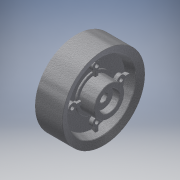
# Autodesk Inventor part: Wheel Hub
Saved by Autodesk Inventor 2018 (Build 220112000, 112)
## iProperties
Created: 2018-08-07
Part Number: Wheel Hub
Material: Generic
Document SubType Name: Modeling
Designer: ruben
Density: 1 g/cm^3
Appearance: Aluminum Cast
Author: ruben
Autodesk Inventor part; units mm, degrees
ref_plane "YZ Plane" through (0, 0, 0) normal (1, 0, 0) x (0, 1, 0)
ref_plane "XZ Plane" through (0, 0, 0) normal (0, 1, 0) x (-1, 0, 0)
ref_plane "XY Plane" through (0, 0, 0) normal (0, 0, 1) x (1, 0, 0)
sketch "Sketch1" plane through (0, 0, 0) normal (0, 1, 0) x (-1, 0, 0)
  line L0 (4.1, 0) -> (-63.1, 0) projected
  line L1 (0, -46.1961) -> (0, 46.6819) projected
  line L2 (-13, -25) -> (-19.5, -25)
  line L3 (-19.5, 25) -> (-13, 25)
  line L4 (-23.9524, -4) -> (-41, -4)
  line L5 (-41, -4) -> (-44, -15)
  line L6 (-23.9524, 4) -> (-41, 4)
  line L7 (-41, 4) -> (-44, 15)
  line L8 (-44, -15) -> (-53.5, -18)
  line L9 (-44, 15) -> (-53.5, 18)
  line L10 (-53.5, -18) -> (-53.5, 18)
  line L11 (-19.5, -25) -> (-19.9524, -6)
  line L12 (-19.9524, 6) -> (-19.5, 25)
  line L13 (-5.5, -16.9) -> (-5.5, 16.9)
  line L14 (-13, -16.9) -> (-5.5, -16.9)
  line L15 (-5.5, 16.9) -> (-13, 16.9)
  line L16 (-13, -25) -> (-13, -16.9)
  line L17 (-13, 16.9) -> (-13, 25)
  line L18 (-44, -26.4766) -> (-44, 27.3254) construction
  line L19 (-19.5, -32.9278) -> (-19.5, 33.4136) construction
  line L20 (-19.9524, -6) -> (-23.9524, -6)
  line L21 (-23.9524, -6) -> (-23.9524, -4)
  line L22 (-23.9524, 4) -> (-23.9524, 6)
  line L23 (-23.9524, 6) -> (-19.9524, 6)
  line L24 (-19.9524, -10.0767) -> (-19.9524, 10.6665) construction
  dimension "d0" = 50
  dimension "d14" = 3
  dimension "d15" = 3
  dimension "d18" = 11
  dimension "d19" = 33.8
  dimension "d36" = 26
  dimension "d48" = 21
  dimension "d49" = 107
  dimension "d50" = 88
  dimension "d52" = 39
  dimension "d53" = 7
  dimension "d54" = 4
  dimension "d56" = 2
  dimension "d57" = 2
  dimension "d58" = 4
  dimension "d60" = 21.0476
  dimension "d61" = 39.9048
  constraints: 46 end point, 10 parallel, 6 point on line, 4 perpendicular, 4 vertical, 2 symmetric about line, 1 collinear, 1 horizontal, 3 other
  measures "d0" distance of L2.start L3.end
  measures "d14" vertical distance of L7.end L9.end
  measures "d15" vertical distance of L5.end L8.end
  measures "d18" diameter of L13 L1
  measures "d19" distance between parallel lines of L15 L14
  measures "d36" diameter of L16 L1
  measures "d48" distance between parallel lines of L4 L2
  measures "d49" diameter of L10 L1
  measures "d50" diameter of L18 L1
  measures "d52" diameter of L19 L1
  measures "d53" distance from line of L2 L8.end
  measures "d54" distance of L11.end L20.end
  measures "d56" distance between parallel lines of L4 L20
  measures "d57" distance of L6.start L22.end
  measures "d58" distance of L12.start L22.end
  measures "d60" horizontal distance of L4.end L11.end
  measures "d61" diameter of L24 L1
revolve "Revolution1" add sketch "Sketch1" angle 360 about axis through (0, 0, -10) along (0, 0, 1)
chamfer "Chamfer1" distance 0.5 angle 45 12 edges at (-19.5, 0, 25) (-13, 0, 25) (-44, 0, 15) (-53.5, 0, 18) (-53.5, 0, -18) (-19.5, 0, -25) (-13, 0, -25) (-5.5, 0, -16.9) (-5.5, 0, 16.9) (-23.9524, 0, 6) (-44, 0, -15) (-23.9524, 0, -6)
sketch "Sketch3" plane through (0, 0, 4) normal (0, 0, 1) x (1, 0, 0)
  line L0 (-74.9, 0) -> (74.9, 0) projected
  line L1 (0, -74.9) -> (0, 74.9) projected
  point P0 (0, 0)
  point P1 (0, 31.5)
  dimension "d25" = 31.5
  constraints: 1 point on line
  measures "d25" distance of point (0, 31.5) point (0, 0)
hole "Hole1" at (0, 31.5, 4) direction (0, 0, -1) diameter 5 end through all
pattern_circular "Circular Pattern1" count 4 over 360 about axis through (0, 0, -10) along (0, 0, 1) of "Hole1"
sketch "Sketch5" plane through (0, 0, 4) normal (0, 0, 1) x (1, 0, 0)
  line L0 (-74.9, 0) -> (74.9, 0) projected
  line L1 (0, -74.9) -> (0, 74.9) projected
  circle A0 centre (0, 0) radius 31.5 construction
  circle A1 centre (0, 31.5) radius 2.5
  line L2 (-2, 36.6235) -> (-2, 44.4318)
  line L3 (2, 36.6235) -> (2, 44.4318)
  circle A2 centre (0, 0) radius 41 projected
  line L4 (-2, 26.3765) -> (-2, 19.8519)
  circle A3 centre (0, 0) radius 23.9524 projected
  line L5 (2, 26.3765) -> (2, 19.8519)
  arc A4 (-2, 36.6235) -> (-2, 26.3765) centre (0, 31.5) ccw
  arc A5 (2, 26.3765) -> (2, 36.6235) centre (0, 31.5) ccw
  circle A6 centre (0, 0) radius 19.9524 projected
  circle A7 centre (0, 0) radius 44.4768 projected
  dimension "d69" = 63
  dimension "d70" = 5
  dimension "d73" = 4
  dimension "d74" = 4
  dimension "d75" = 36.6235
  constraints: 8 end point, 8 point on circle, 3 centre point, 2 coincident, 2 vertical, 1 point on line, 1 symmetric about line, 1 vertical alignment, 4 other
  measures "d70" diameter of A1
  measures "d73" distance between parallel lines of L5 L4
  measures "d74" distance between parallel lines of L3 L2
  measures "d75" vertical distance of A2.centre L3.start
extrude "Extrusion2" add sketch "Sketch5" along normal blind 5 contours A6 L1 A3 L5 | A3 L1 A1 A2 L3 A5 L5 | A6 L4 A3 L1 | A2 L1 A7 L3 | A3 L4 A4 L2 A2 L1 A1 | A2 L2 A7 L1
pattern_circular "Circular Pattern2" count 4 over 360 about axis through (0, 0, -10) along (0, 0, 1) of "Extrusion2"
mirror "Mirror1" about plane through (0, 0, 0) normal (0, 0, 1) of "Extrusion2", "Circular Pattern2"
fillet "Fillet2" radius 0.5 48 edges at (-31.5, 5.5, 9) (-39.4699, 2, 9) (-39.4699, -2, 9) (-31.5, -5.5, 9) (-23.1142, -2, 9) (-23.1142, 2, 9) (2, -23.1142, 9) (-2, -23.1142, 9) (-5.5, -31.5, 9) (-2, -39.4699, 9) (2, -39.4699, 9) (5.5, -31.5, 9) (23.1142, -2, 9) (23.1142, 2, 9) (31.5, 5.5, 9) (31.5, -5.5, 9) (39.4699, -2, 9) (39.4699, 2, 9) (2, 23.1142, 9) (-2, 23.1142, 9) (-5.5, 31.5, 9) (5.5, 31.5, 9) (-2, 39.4699, 9) (2, 39.4699, 9) (2, 23.1142, -9) (-2, 23.1142, -9) (5.5, 31.5, -9) (-5.5, 31.5, -9) (2, 39.4699, -9) (-2, 39.4699, -9) (-23.1142, 2, -9) (-23.1142, -2, -9) (-31.5, -5.5, -9) (-31.5, 5.5, -9) (-39.4699, -2, -9) (-39.4699, 2, -9) (2, -39.4699, -9) (-2, -39.4699, -9) (-5.5, -31.5, -9) (5.5, -31.5, -9) (2, -23.1142, -9) (-2, -23.1142, -9) (39.4699, -2, -9) (39.4699, 2, -9) (31.5, -5.5, -9) (31.5, 5.5, -9) (23.1142, 2, -9) (23.1142, -2, -9)
equation "\"d14\" = d15"
body "Solid1"
